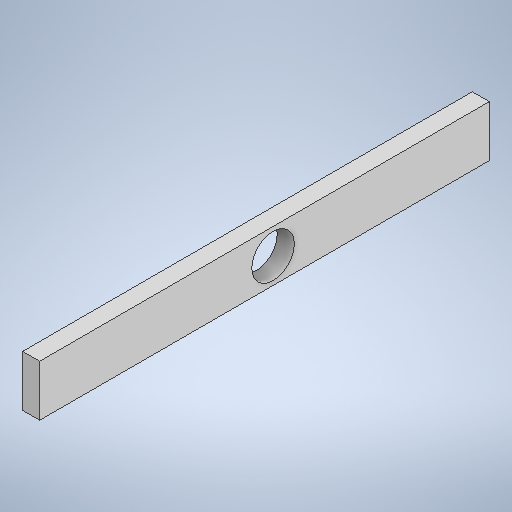
# Autodesk Inventor part: exHelice
Saved by Autodesk Inventor 2025 (Build 290162000, 162)
## iProperties
Created: 2025-04-04
Part Number: exHelice
Material: Genérico
Document SubType Name: Modeling
Designer: Ian
Density: 1 g/cm^3
Appearance: Padrão
Author: Ian
Autodesk Inventor part; units mm, degrees
ref_plane "YZ Plane" through (0, 0, 0) normal (1, 0, 0) x (0, 1, 0)
ref_plane "XZ Plane" through (0, 0, 0) normal (0, 1, 0) x (-1, 0, 0)
ref_plane "XY Plane" through (0, 0, 0) normal (0, 0, 1) x (1, 0, 0)
sketch "Esboço1" plane through (0, 0, 0) normal (0, 1, 0) x (-1, 0, 0)
  line L0 (-5, 132) -> (5, 132)
  line L1 (5, 132) -> (5, -132)
  line L2 (5, -132) -> (-5, -132)
  line L3 (-5, -132) -> (-5, 132)
  line L4 (-5, 132) -> (5, -132) construction
  line L5 (5, 132) -> (-5, -132) construction
  point P0 (0, 0)
  dimension "d0" = 264
  dimension "d1" = 10
  constraints: 12 end point, 2 midpoint, 2 parallel, 1 horizontal, 1 perpendicular
  measures "d0" distance of L0.end L1.end
  measures "d1" distance of L0.start L0.end
extrude "Extrusão1" add sketch "Esboço1" along normal blind 30
sketch "Esboço2" plane through (0, 0, 0) normal (0, -1, 0) x (1, 0, 0)
  point P0 (0, 0)
sketch "Esboço3" plane through (5, 0, 132) normal (1, 0, 0) x (0, 0, -1)
  line L0 (264, 30) -> (0, 30) projected
  circle A0 centre (137, 15) radius 12.5
  line L1 (0, 0) -> (264, 0) projected
  line L2 (264, 0) -> (264, 30) projected
  point P0 (132, 0)
  point P1 (132, 0)
  dimension "d4" = 25
  dimension "d6" = 127
  dimension "d7" = 15
  constraints: 1 centre point, 1 midpoint
  measures "d4" diameter of A0
  measures "d6" distance from line of L2 A0.centre
  measures "d7" distance from line of L1 A0.centre
extrude "Extrusão2" cut sketch "Esboço3" against normal blind 30
